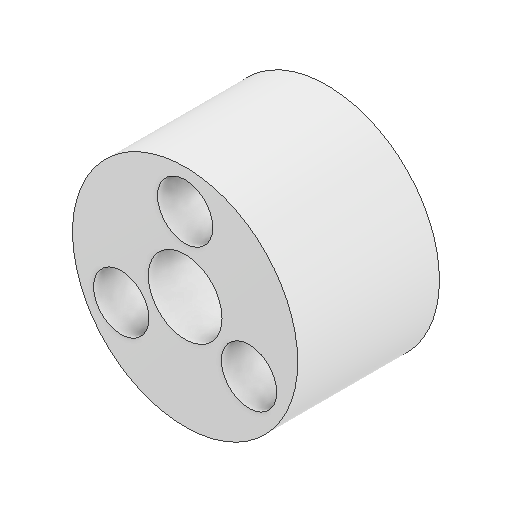
# Autodesk Inventor part: ScissorPin
Saved by Autodesk Inventor 2026.2 (Build 302298000, 298)
## iProperties
Created: 2026-03-23
Part Number: ScissorPin
Material: ABS Plastic
Document SubType Name: Modeling
Designer: gaoet
Density: 1.06 g/cm^3
Appearance: Smooth - White
Author: gaoet
Autodesk Inventor part; units mm, degrees
ref_plane "YZ Plane" through (0, 0, 0) normal (1, 0, 0) x (0, 1, 0)
ref_plane "XZ Plane" through (0, 0, 0) normal (0, 1, 0) x (-1, 0, 0)
ref_plane "XY Plane" through (0, 0, 0) normal (0, 0, 1) x (1, 0, 0)
sketch "Sketch1" plane through (0, 0, 0) normal (0, 0, 1) x (1, 0, 0)
  circle A0 centre (0, 0) radius 6.1
  dimension "d0" = 12.2
  constraints: 1 centre point, 1 coincident
  measures "d0" diameter of A0
extrude "Extrusion1" add sketch "Sketch1" along normal blind 7.68
sketch "Sketch2" plane through (0, 0, 7.68) normal (0, 0, 1) x (1, 0, 0)
  circle A0 centre (0, 0) radius 6.1 projected
  line L0 (0, 4) -> (0, 0) construction
  line L1 (0, 0) -> (-3.4641, -2) construction
  line L2 (3.4641, -2) -> (0, 0) construction
  dimension "d3" = 120
  dimension "d4" = 120
  dimension "d5" = 4
  constraints: 6 end point, 2 equal length, 1 vertical, 1 vertical alignment
  measures "d3" angle of L1 L0
  measures "d4" angle of L2 L0
  measures "d5" distance of L2.start L0.end
hole "Hole1" at (0, 4, 7.68) at (-3.4641, -2, 7.68) at (3.4641, -2, 7.68) direction (0, 0, -1) diameter 3 depth 7
sketch "Sketch3" plane through (0, 0, 0) normal (0, 0, -1) x (-1, 0, 0)
  point P0 (0, 0)
hole "Hole2" at (0, 0, 0) direction (0, 0, 1) diameter 4 end through all
equation "\"d4\" = d3"
body "Solid1"
